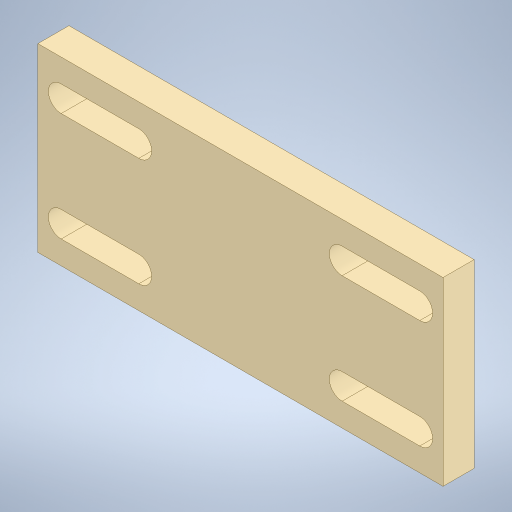
# Autodesk Inventor part: стена_каретка
Saved by Autodesk Inventor 2023.1 (Build 271208000, 208)
## iProperties
Created: 2026-02-21
Part Number: стена_каретка
Material: Типовые
Document SubType Name: Modeling
Designer: DELL
Density: 1 g/cm^3
Appearance: Бежевый
Author: DELL
Autodesk Inventor part; units mm, degrees
ref_plane "YZ Plane" through (0, 0, 0) normal (1, 0, 0) x (0, 1, 0)
ref_plane "XZ Plane" through (0, 0, 0) normal (0, 1, 0) x (-1, 0, 0)
ref_plane "XY Plane" through (0, 0, 0) normal (0, 0, 1) x (1, 0, 0)
sketch "Эскиз1" plane through (0, 0, 0) normal (0, 0, 1) x (1, 0, 0)
  line L0 (-13.1, -7) -> (13.1, -7) construction
  line L1 (13.1, -7) -> (13.1, 7) construction
  line L2 (13.1, 7) -> (-13.1, 7) construction
  line L3 (-13.1, 7) -> (-13.1, -7) construction
  line L4 (-13.1, -7) -> (13.1, 7) construction
  line L5 (13.1, -7) -> (-13.1, 7) construction
  line L6 (13.1, 7) -> (23.1, 7) construction
  line L7 (13.1, 5.35) -> (23.1, 5.35)
  line L8 (23.1, 8.65) -> (13.1, 8.65)
  arc A0 (13.1, 8.65) -> (13.1, 5.35) centre (13.1, 7) ccw
  arc A1 (23.1, 5.35) -> (23.1, 8.65) centre (23.1, 7) ccw
  line L9 (-26.1, -11.65) -> (26.1, -11.65)
  line L10 (26.1, -11.65) -> (26.1, 11.65)
  line L11 (26.1, 11.65) -> (-26.1, 11.65)
  line L12 (-26.1, 11.65) -> (-26.1, -11.65)
  line L13 (-26.1, -11.65) -> (26.1, 11.65) construction
  line L14 (26.1, -11.65) -> (-26.1, 11.65) construction
  line L15 (0, 0) -> (0, -11.65)
  line L16 (0, 0) -> (26.1, 0)
  line L17 (13.1, -5.35) -> (23.1, -5.35)
  line L18 (23.1, -8.65) -> (13.1, -8.65)
  arc A2 (13.1, -5.35) -> (13.1, -8.65) centre (13.1, -7) ccw
  arc A3 (23.1, -8.65) -> (23.1, -5.35) centre (23.1, -7) ccw
  line L19 (-13.1, 7) -> (-23.1, 7) construction
  line L20 (-13.1, 5.35) -> (-23.1, 5.35)
  line L21 (-23.1, 8.65) -> (-13.1, 8.65)
  arc A4 (-13.1, 5.35) -> (-13.1, 8.65) centre (-13.1, 7) ccw
  arc A5 (-23.1, 8.65) -> (-23.1, 5.35) centre (-23.1, 7) ccw
  line L22 (-13.1, -5.35) -> (-23.1, -5.35)
  arc A6 (-13.1, -8.65) -> (-13.1, -5.35) centre (-13.1, -7) ccw
  line L23 (-23.1, -8.65) -> (-13.1, -8.65)
  arc A7 (-23.1, -5.35) -> (-23.1, -8.65) centre (-23.1, -7) ccw
  point P0 (18.1, 7)
  point P1 (-18.1, 7)
  dimension "d0" = 14
  dimension "d1" = 26.2
  dimension "d2" = 10
  dimension "d3" = 3.3
  dimension "d4" = 3
  dimension "d5" = 3
  constraints: 52 end point, 16 point on circle, 16 symmetric about line, 8 centre point, 7 midpoint, 5 parallel, 4 tangent, 3 horizontal, 2 perpendicular, 6 other
  measures "d0" distance of L2.end L0.start
  measures "d1" distance of L1.end L2.end
  measures "d2" distance of L1.end L6.end
  measures "d3" diameter of A1
  measures "d4" distance from line of L10 A3.centre
  measures "d5" distance between parallel lines of L11 L8
extrude "Выдавливание1" add sketch "Эскиз1" along normal blind 4
